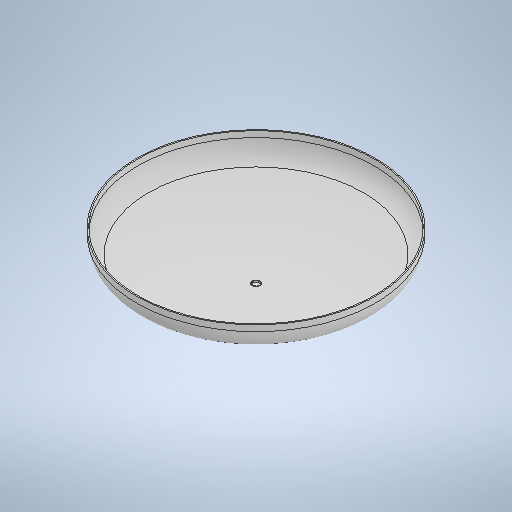
# Autodesk Inventor part: PRS 1604 dished head_D1200
Saved by Autodesk Inventor 2026.2 (Build 302298000, 298)
## iProperties
Created: 2025-02-16
Part Number: PRS 1604 dished head_D1200
Material: Generic
Document SubType Name: Modeling
Designer: admin
Density: 1 g/cm^3
Appearance: Default
Author: pokla
Autodesk Inventor part; units mm, degrees
ref_plane "YZ Plane" through (0, 0, 0) normal (1, 0, 0) x (0, 1, 0)
ref_plane "XZ Plane" through (0, 0, 0) normal (0, 1, 0) x (-1, 0, 0)
ref_plane "XY Plane" through (0, 0, 0) normal (0, 0, 1) x (1, 0, 0)
sketch "Sketch1" plane through (0, 0, 0) normal (0, 1, 0) x (-1, 0, 0)
  line L0 (600, 0) -> (600, -30)
  arc A0 (542.1993, -124.4078) -> (600, -30) centre (494, -30) ccw
  arc A1 (20, -250) -> (542.1993, -124.4078) centre (20, 898.4211) ccw
  line L1 (0, 0) -> (0, -191.6842)
  arc A2 (20, -244) -> (539.4711, -119.0639) centre (20, 898.4211) ccw
  arc A3 (539.4711, -119.0639) -> (594, -30) centre (494, -30) ccw
  line L2 (594, -30) -> (594, 0)
  line L3 (594, 0) -> (600, 0)
  line L4 (0, -244) -> (0, -250)
  line L5 (0, -250) -> (20, -250)
  line L6 (0, -244) -> (20, -244)
  point P0 (0, 0)
  point P1 (0, -163.7009)
  point P2 (0, -169.7009)
  dimension "d1" = 30
  dimension "d3" = 1148.421
  dimension "d11" = 1188
  dimension "d12" = 250
  dimension "d13" = 6
  dimension "d14" = 40
  dimension "d15" = 100
  constraints: 14 end point, 8 point on circle, 4 centre point, 3 horizontal, 3 tangent, 2 vertical, 1 coincident, 1 horizontal alignment, 1 parallel, 1 perpendicular, 1 point on line, 1 vertical alignment, 1 other
  measures "d1" distance of L0.start L0.end
  measures "d3" radius of A1
  measures "d11" diameter of L2 L1
  measures "d12" distance of L4.end point (0, 0)
  measures "d13" distance of L2.end L0.start
  measures "d14" diameter of L5.end L1
  measures "d15" radius of A3
revolve "Revolution1" add sketch "Sketch1" angle 360 about axis through (0, 0, 0) along (0, 0, -1)
sketch "Sketch2" plane through (0, 0, 0) normal (0, 0, 1) x (1, 0, 0)
  circle A0 centre (0, 0) radius 16.75
  dimension "d8" = 33.5
  constraints: 1 centre point, 1 coincident
  measures "d8" diameter of A0
extrude "Extrusion1" cut sketch "Sketch2" against normal through all
body "Solid1"
